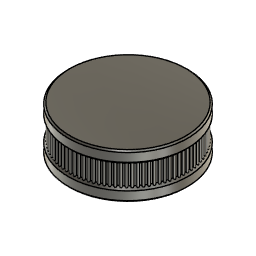
OSSM - Mounting Ring - PitClamp Mini - Parametric (Autodesk Fusion 360 design; units mm, degrees)
Autodesk Fusion 360 part; units mm, degrees
note: some values were not read from the file. Set by a fixed rule: which sketch regions a step uses.
sketch "Sketch1" plane through (0, 0, 0) normal (0, 0, 1) x (1, 0, 0)
  circle A0 centre (0, 0) radius 40
  circle A1 centre (0, 0) radius 38.25
  line L0 (0, 0) -> (0, 38.25)
  circle A2 centre (0, 38.25) radius 0.75
  circle A3 centre (-2.6682, 38.1568) radius 0.75
  circle A4 centre (-5.3234, 37.8778) radius 0.75
  circle A5 centre (-7.9526, 37.4141) radius 0.75
  circle A6 centre (-10.5431, 36.7683) radius 0.75
  circle A7 centre (-13.0823, 35.9432) radius 0.75
  circle A8 centre (-15.5577, 34.9431) radius 0.75
  circle A9 centre (-17.9573, 33.7727) radius 0.75
  circle A10 centre (-20.2694, 32.4378) radius 0.75
  circle A11 centre (-22.4828, 30.9449) radius 0.75
  circle A12 centre (-24.5866, 29.3012) radius 0.75
  circle A13 centre (-26.5707, 27.5147) radius 0.75
  circle A14 centre (-28.4253, 25.5942) radius 0.75
  circle A15 centre (-30.1414, 23.5491) radius 0.75
  circle A16 centre (-31.7107, 21.3891) radius 0.75
  circle A17 centre (-33.1255, 19.125) radius 0.75
  circle A18 centre (-34.3789, 16.7677) radius 0.75
  circle A19 centre (-35.4648, 14.3287) radius 0.75
  circle A20 centre (-36.3779, 11.8199) radius 0.75
  circle A21 centre (-37.1138, 9.2535) radius 0.75
  circle A22 centre (-37.6689, 6.642) radius 0.75
  circle A23 centre (-38.0405, 3.9982) radius 0.75
  circle A24 centre (-38.2267, 1.3349) radius 0.75
  circle A25 centre (-38.2267, -1.3349) radius 0.75
  circle A26 centre (-38.0405, -3.9982) radius 0.75
  circle A27 centre (-37.6689, -6.642) radius 0.75
  circle A28 centre (-37.1138, -9.2535) radius 0.75
  circle A29 centre (-36.3779, -11.8199) radius 0.75
  circle A30 centre (-35.4648, -14.3287) radius 0.75
  circle A31 centre (-34.3789, -16.7677) radius 0.75
  circle A32 centre (-33.1255, -19.125) radius 0.75
  circle A33 centre (-31.7107, -21.3891) radius 0.75
  circle A34 centre (-30.1414, -23.5491) radius 0.75
  circle A35 centre (-28.4253, -25.5942) radius 0.75
  circle A36 centre (-26.5707, -27.5147) radius 0.75
  circle A37 centre (-24.5866, -29.3012) radius 0.75
  circle A38 centre (-22.4828, -30.9449) radius 0.75
  circle A39 centre (-20.2694, -32.4378) radius 0.75
  circle A40 centre (-17.9573, -33.7727) radius 0.75
  circle A41 centre (-15.5577, -34.9431) radius 0.75
  circle A42 centre (-13.0823, -35.9432) radius 0.75
  circle A43 centre (-10.5431, -36.7683) radius 0.75
  circle A44 centre (-7.9526, -37.4141) radius 0.75
  circle A45 centre (-5.3234, -37.8778) radius 0.75
  circle A46 centre (-2.6682, -38.1568) radius 0.75
  circle A47 centre (0, -38.25) radius 0.75
  circle A48 centre (2.6682, -38.1568) radius 0.75
  circle A49 centre (5.3234, -37.8778) radius 0.75
  circle A50 centre (7.9526, -37.4141) radius 0.75
  circle A51 centre (10.5431, -36.7683) radius 0.75
  circle A52 centre (13.0823, -35.9432) radius 0.75
  circle A53 centre (15.5577, -34.9431) radius 0.75
  circle A54 centre (17.9573, -33.7727) radius 0.75
  circle A55 centre (20.2694, -32.4378) radius 0.75
  circle A56 centre (22.4828, -30.9449) radius 0.75
  circle A57 centre (24.5866, -29.3012) radius 0.75
  circle A58 centre (26.5707, -27.5147) radius 0.75
  circle A59 centre (28.4253, -25.5942) radius 0.75
  circle A60 centre (30.1414, -23.5491) radius 0.75
  circle A61 centre (31.7107, -21.3891) radius 0.75
  circle A62 centre (33.1255, -19.125) radius 0.75
  circle A63 centre (34.3789, -16.7677) radius 0.75
  circle A64 centre (35.4648, -14.3287) radius 0.75
  circle A65 centre (36.3779, -11.8199) radius 0.75
  circle A66 centre (37.1138, -9.2535) radius 0.75
  circle A67 centre (37.6689, -6.642) radius 0.75
  circle A68 centre (38.0405, -3.9982) radius 0.75
  circle A69 centre (38.2267, -1.3349) radius 0.75
  circle A70 centre (38.2267, 1.3349) radius 0.75
  circle A71 centre (38.0405, 3.9982) radius 0.75
  circle A72 centre (37.6689, 6.642) radius 0.75
  circle A73 centre (37.1138, 9.2535) radius 0.75
  circle A74 centre (36.3779, 11.8199) radius 0.75
  circle A75 centre (35.4648, 14.3287) radius 0.75
  circle A76 centre (34.3789, 16.7677) radius 0.75
  circle A77 centre (33.1255, 19.125) radius 0.75
  circle A78 centre (31.7107, 21.3891) radius 0.75
  circle A79 centre (30.1414, 23.5491) radius 0.75
  circle A80 centre (28.4253, 25.5942) radius 0.75
  circle A81 centre (26.5707, 27.5147) radius 0.75
  circle A82 centre (24.5866, 29.3012) radius 0.75
  circle A83 centre (22.4828, 30.9449) radius 0.75
  circle A84 centre (20.2694, 32.4378) radius 0.75
  circle A85 centre (17.9573, 33.7727) radius 0.75
  circle A86 centre (15.5577, 34.9431) radius 0.75
  circle A87 centre (13.0823, 35.9432) radius 0.75
  circle A88 centre (10.5431, 36.7683) radius 0.75
  circle A89 centre (7.9526, 37.4141) radius 0.75
  circle A90 centre (5.3234, 37.8778) radius 0.75
  circle A91 centre (2.6682, 38.1568) radius 0.75
  dimension "d7" = 80
  dimension "d20" = 1.5
  dimension "d23" = 360
  constraint coincident A0.centre A1.centre
  constraint coincident A1 L0.end
  constraint vertical L0
  constraint coincident L0.end A2.centre
  measures "d7" diameter of A0
  measures "d20" diameter of A2
extrude "Extrude1" add sketch "Sketch1" along normal blind 6.7 contours A0 | A1 A2 A3 A4 A5 A6 A7 A8 A9 A10 A11 A12 A13 A14 A15 A16 A17 A18 A19 A20 A21 A22 A23 A24 A25 A26 A27 A28 A29 A30 A31 A32 A33 A34 A35 A36 A37 A38 A39 A40 A41 A42 A43 A44 A45 A46 A47 A48 A49 A50 A51 A52 A53 A54 A55 A56 A57 A58 A59 A60 A61 A62 A63 A64 A65 A66 A67 A68 A69 A70 A71 A72 A73 A74 A75 A76 A77 A78 A79 A80 A81 A82 A83 A84 A85 A86 A87 A88 A89 A90 A91 | A1 A70 | A1 A70 | A1 A69 | A1 A69 | A1 A71 | A1 A71 | A1 A68 | A1 A68 | A1 A72 | A1 A72 | A1 A67 | A1 A67 | A1 A73 | A1 A73 | A1 A66 | A1 A66 | A1 A74 | A1 A74 | A1 A65 | A1 A65 | A1 A75 | A1 A75 | A1 A64 | A1 A64 | A1 A76 | A1 A76 | A1 A63 | A1 A63 | A1 A77 | A1 A77 | A1 A62 | A1 A62 | A1 A78 | A1 A78 | A1 A61 | A1 A61 | A1 A79 | A1 A79 | A1 A60 | A1 A60 | A1 A80 | A1 A80 | A1 A59 | A1 A59 | A1 A81 | A1 A81 | A1 A58 | A1 A58 | A1 A82 | A1 A82 | A1 A57 | A1 A57 | A1 A83 | A1 A83 | A1 A56 | A1 A56 | A1 A84 | A1 A84 | A1 A55 | A1 A55 | A1 A85 | A1 A85 | A1 A54 | A1 A54 | A1 A86 | A1 A86 | A1 A53 | A1 A53 | A1 A87 | A1 A87 | A1 A52 | A1 A52 | A1 A88 | A1 A88 | A1 A51 | A1 A51 | A1 A89 | A1 A89 | A1 A50 | A1 A50 | A1 A90 | A1 A90 | A1 A49 | A1 A49 | A1 A91 | A1 A91 | A1 A48 | A1 A48 | A1 L0 A2 | A1 A2 | A1 A47 | A1 A47 | A1 L0 A2 | A1 A46 | A1 A46 | A1 A3 | A1 A3 | A1 A45 | A1 A45 | A1 A4 | A1 A4 | A1 A44 | A1 A44 | A1 A5 | A1 A5 | A1 A43 | A1 A43 | A1 A6 | A1 A6 | A1 A42 | A1 A42 | A1 A7 | A1 A7 | A1 A41 | A1 A41 | A1 A8 | A1 A8 | A1 A40 | A1 A40 | A1 A9 | A1 A9 | A1 A39 | A1 A39 | A1 A10 | A1 A10 | A1 A38 | A1 A38 | A1 A11 | A1 A11 | A1 A37 | A1 A37 | A1 A12 | A1 A12 | A1 A36 | A1 A36 | A1 A13 | A1 A13 | A1 A35 | A1 A35 | A1 A14 | A1 A14 | A1 A34 | A1 A34 | A1 A15 | A1 A15 | A1 A33 | A1 A33 | A1 A16 | A1 A16 | A1 A32 | A1 A32 | A1 A17 | A1 A17 | A1 A31 | A1 A31 | A1 A18 | A1 A18 | A1 A30 | A1 A30 | A1 A19 | A1 A19 | A1 A29 | A1 A29 | A1 A20 | A1 A20 | A1 A28 | A1 A28 | A1 A21 | A1 A21 | A1 A27 | A1 A27 | A1 A22 | A1 A22 | A1 A26 | A1 A26 | A1 A23 | A1 A23 | A1 A25 | A1 A25 | A1 A24 | A1 A24 makes body 1
extrude "Extrude2" add sketch "Sketch1" along normal blind 6.7 from surface at 23.3 separate body contours A0 | A1 A2 A3 A4 A5 A6 A7 A8 A9 A10 A11 A12 A13 A14 A15 A16 A17 A18 A19 A20 A21 A22 A23 A24 A25 A26 A27 A28 A29 A30 A31 A32 A33 A34 A35 A36 A37 A38 A39 A40 A41 A42 A43 A44 A45 A46 A47 A48 A49 A50 A51 A52 A53 A54 A55 A56 A57 A58 A59 A60 A61 A62 A63 A64 A65 A66 A67 A68 A69 A70 A71 A72 A73 A74 A75 A76 A77 A78 A79 A80 A81 A82 A83 A84 A85 A86 A87 A88 A89 A90 A91 | A1 A70 | A1 A70 | A1 A69 | A1 A69 | A1 A71 | A1 A71 | A1 A68 | A1 A68 | A1 A72 | A1 A72 | A1 A67 | A1 A67 | A1 A73 | A1 A73 | A1 A66 | A1 A66 | A1 A74 | A1 A74 | A1 A65 | A1 A65 | A1 A75 | A1 A75 | A1 A64 | A1 A64 | A1 A76 | A1 A76 | A1 A63 | A1 A63 | A1 A77 | A1 A77 | A1 A62 | A1 A62 | A1 A78 | A1 A78 | A1 A61 | A1 A61 | A1 A79 | A1 A79 | A1 A60 | A1 A60 | A1 A80 | A1 A80 | A1 A59 | A1 A59 | A1 A81 | A1 A81 | A1 A58 | A1 A58 | A1 A82 | A1 A82 | A1 A57 | A1 A57 | A1 A83 | A1 A83 | A1 A56 | A1 A56 | A1 A84 | A1 A84 | A1 A55 | A1 A55 | A1 A85 | A1 A85 | A1 A54 | A1 A54 | A1 A86 | A1 A86 | A1 A53 | A1 A53 | A1 A87 | A1 A87 | A1 A52 | A1 A52 | A1 A88 | A1 A88 | A1 A51 | A1 A51 | A1 A89 | A1 A89 | A1 A50 | A1 A50 | A1 A90 | A1 A90 | A1 A49 | A1 A49 | A1 A91 | A1 A91 | A1 A48 | A1 A48 | A1 L0 A2 | A1 A2 | A1 A47 | A1 A47 | A1 L0 A2 | A1 A46 | A1 A46 | A1 A3 | A1 A3 | A1 A45 | A1 A45 | A1 A4 | A1 A4 | A1 A44 | A1 A44 | A1 A5 | A1 A5 | A1 A43 | A1 A43 | A1 A6 | A1 A6 | A1 A42 | A1 A42 | A1 A7 | A1 A7 | A1 A41 | A1 A41 | A1 A8 | A1 A8 | A1 A40 | A1 A40 | A1 A9 | A1 A9 | A1 A39 | A1 A39 | A1 A10 | A1 A10 | A1 A38 | A1 A38 | A1 A11 | A1 A11 | A1 A37 | A1 A37 | A1 A12 | A1 A12 | A1 A36 | A1 A36 | A1 A13 | A1 A13 | A1 A35 | A1 A35 | A1 A14 | A1 A14 | A1 A34 | A1 A34 | A1 A15 | A1 A15 | A1 A33 | A1 A33 | A1 A16 | A1 A16 | A1 A32 | A1 A32 | A1 A17 | A1 A17 | A1 A31 | A1 A31 | A1 A18 | A1 A18 | A1 A30 | A1 A30 | A1 A19 | A1 A19 | A1 A29 | A1 A29 | A1 A20 | A1 A20 | A1 A28 | A1 A28 | A1 A21 | A1 A21 | A1 A27 | A1 A27 | A1 A22 | A1 A22 | A1 A26 | A1 A26 | A1 A23 | A1 A23 | A1 A25 | A1 A25 | A1 A24 | A1 A24 makes body 2
extrude "Extrude3" add sketch "Sketch1" along normal blind 16.6 from surface at 6.7 contours A1 A2 A3 A4 A5 A6 A7 A8 A9 A10 A11 A12 A13 A14 A15 A16 A17 A18 A19 A20 A21 A22 A23 A24 A25 A26 A27 A28 A29 A30 A31 A32 A33 A34 A35 A36 A37 A38 A39 A40 A41 A42 A43 A44 A45 A46 A47 A48 A49 A50 A51 A52 A53 A54 A55 A56 A57 A58 A59 A60 A61 A62 A63 A64 A65 A66 A67 A68 A69 A70 A71 A72 A73 A74 A75 A76 A77 A78 A79 A80 A81 A82 A83 A84 A85 A86 A87 A88 A89 A90 A91 | A1 A70 | A1 A69 | A1 A71 | A1 A68 | A1 A72 | A1 A67 | A1 A73 | A1 A66 | A1 A74 | A1 A65 | A1 A75 | A1 A64 | A1 A76 | A1 A63 | A1 A77 | A1 A62 | A1 A78 | A1 A61 | A1 A79 | A1 A60 | A1 A80 | A1 A59 | A1 A81 | A1 A58 | A1 A82 | A1 A57 | A1 A83 | A1 A56 | A1 A84 | A1 A55 | A1 A85 | A1 A54 | A1 A86 | A1 A53 | A1 A87 | A1 A52 | A1 A88 | A1 A51 | A1 A89 | A1 A50 | A1 A90 | A1 A49 | A1 A91 | A1 A48 | A1 L0 A2 | A1 A47 | A1 L0 A2 | A1 A46 | A1 A3 | A1 A45 | A1 A4 | A1 A44 | A1 A5 | A1 A43 | A1 A6 | A1 A42 | A1 A7 | A1 A41 | A1 A8 | A1 A40 | A1 A9 | A1 A39 | A1 A10 | A1 A38 | A1 A11 | A1 A37 | A1 A12 | A1 A36 | A1 A13 | A1 A35 | A1 A14 | A1 A34 | A1 A15 | A1 A33 | A1 A16 | A1 A32 | A1 A17 | A1 A31 | A1 A18 | A1 A30 | A1 A19 | A1 A29 | A1 A20 | A1 A28 | A1 A21 | A1 A27 | A1 A22 | A1 A26 | A1 A23 | A1 A25 | A1 A24 picked at (37.9776, 1.3076) picked at (37.9763, -1.3447) picked at (37.79, 3.9906) picked at (37.79, -3.9906) picked at (37.4196, 6.6169) picked at (37.4261, -6.5804) picked at (36.8669, 9.2111) picked at (36.8759, -9.1751) picked at (36.1345, 11.7603) picked at (36.1345, -11.7603) picked at (35.2401, 14.2179) picked at (35.2262, -14.2523) picked at (34.1462, 16.6749) picked at (34.1462, -16.6749) picked at (32.9184, 18.984) picked at (32.9184, -18.984) picked at (31.4932, 21.2648) picked at (31.4932, -21.2648) picked at (29.9331, 23.4099) picked at (29.9331, -23.4099) picked at (28.2272, 25.4409) picked at (28.2272, -25.4409) picked at (26.4105, 27.3221) picked at (26.3838, -27.3479) picked at (24.4402, 29.0979) picked at (24.4118, -29.1217) picked at (22.3509, 30.7319) picked at (22.3209, -30.7537) picked at (20.1528, 32.2161) picked at (20.1213, -32.2358) picked at (17.8236, 33.5609) picked at (17.8236, -33.5609) picked at (15.4391, 34.7224) picked at (15.4391, -34.7224) picked at (12.9794, 35.7148) picked at (13.0143, -35.7021) picked at (10.4564, 36.5332) picked at (10.4564, -36.5332) picked at (7.9188, 37.1659) picked at (7.9188, -37.1659) picked at (5.307, 37.6277) picked at (5.2702, -37.6329) picked at (2.6322, 37.9089) picked at (2.6322, -37.9089) picked at (0.0186, -38.0001) picked at (-2.64, -37.9079) picked at (-2.64, 37.9079) picked at (-5.3046, -37.6279) picked at (-5.3046, 37.6279) picked at (-7.8893, -37.1717) picked at (-7.8893, 37.1717) picked at (-10.4722, -36.528) picked at (-10.4722, 36.528) picked at (-12.9849, -35.7124) picked at (-12.9849, 35.7124) picked at (-15.4536, -34.7152) picked at (-15.4536, 34.7152) picked at (-17.8279, -33.5582) picked at (-17.8279, 33.5582) picked at (-20.1342, -32.2269) picked at (-20.1342, 32.2269) picked at (-22.3239, -30.7512) picked at (-22.3239, 30.7512) picked at (-24.423, -29.1115) picked at (-24.423, 29.1115) picked at (-26.3855, -27.346) picked at (-26.3855, 27.346) picked at (-28.2364, -25.4296) picked at (-28.2364, 25.4296) picked at (-29.9337, -23.409) picked at (-29.9337, 23.409) picked at (-31.5004, -21.253) picked at (-31.5004, 21.253) picked at (-32.918, -18.9845) picked at (-32.918, 18.9845) picked at (-34.1513, -16.6628) picked at (-34.1513, 16.6628) picked at (-35.239, -14.22) picked at (-35.239, 14.22) picked at (-36.1377, -11.7486) picked at (-36.1377, 11.7486) picked at (-36.8729, -9.1848) picked at (-36.8729, 9.1848) picked at (-37.421, -6.6059) picked at (-37.421, 6.6059) picked at (-37.7923, -3.9636) picked at (-37.7923, 3.9636) picked at (-37.9762, -1.3349) picked at (-37.9762, 1.3349) bodies 1 2
chamfer "Chamfer1" distance 1.75 angle 45 1 edges at (-35.6615, 13.8318, 6.7) on bodies 1
chamfer "Chamfer2" distance 1.75 angle 45 1 edges at (-35.6615, -13.8318, 23.3) on bodies 1
extrude "Extrude4" add sketch "Sketch1" along normal blind 16.6 from surface at 6.7 contours A1 A70 | A1 A70 | A1 A69 | A1 A69 | A1 A71 | A1 A71 | A1 A68 | A1 A68 | A1 A72 | A1 A72 | A1 A67 | A1 A67 | A1 A73 | A1 A73 | A1 A66 | A1 A66 | A1 A74 | A1 A74 | A1 A65 | A1 A65 | A1 A75 | A1 A75 | A1 A64 | A1 A64 | A1 A76 | A1 A76 | A1 A63 | A1 A63 | A1 A77 | A1 A77 | A1 A62 | A1 A62 | A1 A78 | A1 A78 | A1 A61 | A1 A61 | A1 A79 | A1 A79 | A1 A60 | A1 A60 | A1 A80 | A1 A80 | A1 A59 | A1 A59 | A1 A81 | A1 A81 | A1 A58 | A1 A58 | A1 A82 | A1 A82 | A1 A57 | A1 A57 | A1 A83 | A1 A83 | A1 A56 | A1 A56 | A1 A84 | A1 A84 | A1 A55 | A1 A55 | A1 A85 | A1 A85 | A1 A54 | A1 A54 | A1 A86 | A1 A86 | A1 A53 | A1 A53 | A1 A87 | A1 A87 | A1 A52 | A1 A52 | A1 A88 | A1 A88 | A1 A51 | A1 A51 | A1 A89 | A1 A89 | A1 A50 | A1 A50 | A1 A90 | A1 A90 | A1 A49 | A1 A49 | A1 A91 | A1 A91 | A1 A48 | A1 A48 | A1 L0 A2 | A1 A2 | A1 A47 | A1 A47 | A1 L0 A2 | A1 A46 | A1 A46 | A1 A3 | A1 A3 | A1 A45 | A1 A45 | A1 A4 | A1 A4 | A1 A44 | A1 A44 | A1 A5 | A1 A5 | A1 A43 | A1 A43 | A1 A6 | A1 A6 | A1 A42 | A1 A42 | A1 A7 | A1 A7 | A1 A41 | A1 A41 | A1 A8 | A1 A8 | A1 A40 | A1 A40 | A1 A9 | A1 A9 | A1 A39 | A1 A39 | A1 A10 | A1 A10 | A1 A38 | A1 A38 | A1 A11 | A1 A11 | A1 A37 | A1 A37 | A1 A12 | A1 A12 | A1 A36 | A1 A36 | A1 A13 | A1 A13 | A1 A35 | A1 A35 | A1 A14 | A1 A14 | A1 A34 | A1 A34 | A1 A15 | A1 A15 | A1 A33 | A1 A33 | A1 A16 | A1 A16 | A1 A32 | A1 A32 | A1 A17 | A1 A17 | A1 A31 | A1 A31 | A1 A18 | A1 A18 | A1 A30 | A1 A30 | A1 A19 | A1 A19 | A1 A29 | A1 A29 | A1 A20 | A1 A20 | A1 A28 | A1 A28 | A1 A21 | A1 A21 | A1 A27 | A1 A27 | A1 A22 | A1 A22 | A1 A26 | A1 A26 | A1 A23 | A1 A23 | A1 A25 | A1 A25 | A1 A24 | A1 A24 bodies 1
chamfer "Chamfer3" distance 1 angle 45 2 edges at (-37.2931, -14.4646, 30) (-37.2931, -14.4646, 0) on bodies 1
equation "Ring_OuterDiameter = 80 mm"
equation "Ring_Thickness = 30 mm"
equation "Ridge_Inset = ( 80 mm - 38.25 * 2 mm ) / 2"
equation "Ridge_NotchDiameter = 1.5 mm"
equation "d7 = Ring_OuterDiameter"
equation "Ridge_Width = 16.6 mm"
equation "d9 = ( Ring_Thickness - Ridge_Width ) / 2"
equation "d11 = ( Ring_Thickness - Ridge_Width ) / 2 + Ridge_Width"
equation "d12 = ( Ring_Thickness - Ridge_Width ) / 2"
equation "d14 = -Ridge_Inset"
equation "d15 = ( Ring_Thickness - Ridge_Width ) / 2"
equation "d16 = Ridge_Width"
equation "d18 = Ridge_Inset"
equation "d19 = Ridge_Inset"
equation "Ridge_NotchCount = 90"
equation "d22 = Ridge_NotchCount"
equation "d24 = ( Ring_Thickness - Ridge_Width ) / 2"
equation "d25 = Ridge_Width"
equation "Ring_Chamfer = 1 mm"
equation "d28 = Ring_Chamfer"
equation "d28 = Ring_Chamfer"
